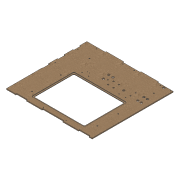
# Autodesk Inventor part: Lateral Derecho Carcasa
Saved by Autodesk Inventor 2020 (Build 240168000, 168)
## iProperties
Created: 2020-06-08
Part Number: Lateral Derecho Carcasa
Material: MDF Tablero de fibras de densidad media
Document SubType Name: Modeling
Designer: Pipi
Density: 0.8 g/cm^3
Appearance: Cartón - Ondulado
Mass: 1380.71 g
Surface Area: 4227.94 cm^2
Volume: 1725.88 cm^3
Author: Pipi
Autodesk Inventor part; units mm, degrees
ref_plane "YZ Plane" through (0, 0, 0) normal (1, 0, 0) x (0, 1, 0)
ref_plane "XZ Plane" through (0, 0, 0) normal (0, 1, 0) x (-1, 0, 0)
ref_plane "XY Plane" through (0, 0, 0) normal (0, 0, 1) x (1, 0, 0)
sketch "Boceto1" plane through (0, 0, 0) normal (0, 1, 0) x (-1, 0, 0)
  line L0 (31.3028, -81.5323) -> (31.3028, -546.5323)
  line L1 (526.8028, -376.5323) -> (521.3028, -376.5323)
  line L2 (521.3028, -326.5323) -> (526.8028, -326.5323)
  line L3 (116.3028, -128.5323) -> (116.3028, -344.5323)
  line L4 (398.303, -351.5323) -> (123.3028, -351.5323)
  line L5 (123.3028, -121.5323) -> (399.3028, -121.5323)
  line L6 (526.8028, -376.5323) -> (526.8028, -326.5323)
  line L7 (521.3028, -416.5323) -> (521.3028, -376.5323)
  line L8 (406.3028, -344.5323) -> (406.3028, -128.5323)
  line L9 (399.3028, -351.5323) -> (123.3028, -351.5323)
  line L10 (123.3028, -121.5323) -> (399.3028, -121.5323)
  arc A0 (399.3028, -351.5323) -> (406.3028, -344.5323) centre (399.3028, -344.5323) ccw
  arc A1 (406.3028, -128.5323) -> (399.3028, -121.5323) centre (399.3028, -128.5323) ccw
  arc A2 (123.3028, -121.5323) -> (116.3028, -128.5323) centre (123.3028, -128.5323) ccw
  arc A3 (116.3028, -344.5323) -> (123.3028, -351.5323) centre (123.3028, -344.5323) ccw
  line L11 (123.3028, -114.5323) -> (399.3028, -114.5323)
  line L12 (413.3028, -128.5323) -> (413.3028, -344.5323)
  line L13 (399.3028, -358.5323) -> (123.3028, -358.5323)
  line L14 (109.3028, -344.5323) -> (109.3028, -128.5323)
  line L15 (109.3028, -128.5323) -> (109.3028, -121.5323)
  line L16 (116.3028, -114.5323) -> (123.3028, -114.5323)
  line L17 (109.3028, -344.5323) -> (109.3028, -351.5323)
  line L18 (116.3028, -358.5323) -> (123.3028, -358.5323)
  line L19 (413.3028, -344.5323) -> (413.3028, -351.5323)
  line L20 (406.3028, -358.5323) -> (399.3028, -358.5323)
  line L21 (413.3028, -128.5323) -> (413.3028, -121.5323)
  line L22 (399.3028, -114.5323) -> (406.3028, -114.5323)
  arc A4 (413.3028, -121.5323) -> (406.3028, -114.5323) centre (406.3028, -121.5323) ccw
  arc A5 (406.3028, -358.5323) -> (413.3028, -351.5323) centre (406.3028, -351.5323) ccw
  arc A6 (109.3028, -351.5323) -> (116.3028, -358.5323) centre (116.3028, -351.5323) ccw
  arc A7 (116.3028, -114.5323) -> (109.3028, -121.5323) centre (116.3028, -121.5323) ccw
  line L23 (421.3028, -552.0323) -> (421.3028, -546.5323)
  line L24 (421.3028, -546.5323) -> (521.3028, -546.5323)
  line L25 (421.3028, -552.0323) -> (321.3028, -552.0323)
  line L26 (321.3028, -552.0323) -> (321.3028, -546.5323)
  line L27 (321.3028, -546.5323) -> (221.3028, -546.5323)
  line L28 (221.3028, -546.5323) -> (221.3028, -552.0323)
  line L29 (319.3028, -81.5323) -> (319.3028, -87.0323)
  line L30 (199.3028, -81.5323) -> (199.3028, -87.0323)
  line L31 (319.3028, -87.0323) -> (199.3028, -87.0323)
  circle A8 centre (76.3028, -156.5323) radius 3
  circle A9 centre (76.3028, -276.5323) radius 3
  line L32 (31.3028, -81.5323) -> (49.3028, -81.5323)
  circle A10 centre (76.3028, -481.0323) radius 3
  line L33 (521.3028, -81.5323) -> (523.8028, -81.5323)
  line L34 (523.8028, -81.5323) -> (523.8028, -286.5323)
  line L35 (523.8028, -286.5323) -> (521.3028, -286.5323)
  line L36 (521.3028, -286.5323) -> (521.3028, -326.5323)
  line L37 (221.3028, -552.0323) -> (121.3028, -552.0323)
  line L38 (121.3028, -552.0323) -> (121.3028, -546.5323)
  line L39 (121.3028, -546.5323) -> (31.3028, -546.5323)
  line L40 (526.8028, -416.5323) -> (521.3028, -416.5323)
  line L41 (526.8028, -416.5323) -> (526.8028, -466.5323)
  line L42 (526.8028, -466.5323) -> (521.3028, -466.5323)
  line L43 (521.3028, -466.5323) -> (521.3028, -506.5323)
  line L44 (521.3028, -506.5323) -> (526.8028, -506.5323)
  line L45 (526.8028, -546.5323) -> (526.8028, -506.5323)
  circle A11 centre (41.0178, -541.5323) radius 2
  circle A12 centre (349.1778, -378.6573) radius 2
  circle A13 centre (386.4278, -378.6573) radius 2
  circle A14 centre (367.8028, -383.8623) radius 2
  line L46 (261.3028, -358.5323) -> (261.3028, -396.5323)
  circle A15 centre (173.4278, -378.6573) radius 2
  circle A16 centre (136.1778, -378.6573) radius 2
  line L47 (521.3028, -546.5323) -> (526.8028, -546.5323)
  circle A17 centre (194.3028, -94.7473) radius 2
  circle A18 centre (324.3028, -94.7473) radius 2
  circle A19 centre (461.8028, -538.0323) radius 2
  circle A20 centre (311.8028, -538.0323) radius 2
  circle A21 centre (96.3028, -538.0323) radius 2
  circle A22 centre (246.3028, -538.0323) radius 2
  circle A23 centre (513.5878, -481.5323) radius 2
  circle A24 centre (513.5878, -351.5323) radius 2
  line L48 (319.3028, -81.5323) -> (409.3028, -81.5323)
  line L49 (409.3028, -81.5323) -> (409.3028, -87.0323)
  line L50 (409.3028, -87.0323) -> (469.3028, -87.0323)
  line L51 (469.3028, -87.0323) -> (469.3028, -81.5323)
  line L52 (521.3028, -81.5323) -> (469.3028, -81.5323)
  line L53 (409.3028, -81.5323) -> (319.3028, -81.5323)
  line L54 (199.3028, -81.5323) -> (109.3028, -81.5323)
  line L55 (109.3028, -81.5323) -> (109.3028, -87.0323)
  line L56 (109.3028, -87.0323) -> (49.3028, -87.0323)
  line L57 (49.3028, -87.0323) -> (49.3028, -81.5323)
  line L58 (31.3028, -81.5323) -> (49.3028, -81.5323)
  line L59 (109.3028, -81.5323) -> (199.3028, -81.5323)
  circle A25 centre (361.8028, -397.5323) radius 1.5
  circle A26 centre (373.8028, -397.5323) radius 1.5
  line L60 (81.3528, -532.0323) -> (70.2528, -532.0323)
  line L61 (70.2528, -532.0323) -> (70.2528, -542.7823)
  line L62 (70.2528, -542.7823) -> (81.3528, -542.7823)
  line L63 (81.3528, -542.7823) -> (81.3528, -532.0323)
  point P0 (0, 0)
  point P1 (398.3028, -355.6989)
  point P2 (109.3028, -358.5323)
  point P3 (413.3028, -358.5323)
  point P4 (413.3028, -114.5323)
  point P5 (398.303, -351.5323)
  dimension "d142" = 230
  dimension "d146" = 85
  dimension "d155" = 5.5
  dimension "d159" = 40
  dimension "d160" = 50
  dimension "d184" = 90
  dimension "d185" = 90
  dimension "d207" = 7
  dimension "d208" = 290
  dimension "d219" = 7
  dimension "d220" = 7
  dimension "d221" = 7
  dimension "d223" = 7
  dimension "d230" = 5.5
  dimension "d235" = 100
  dimension "d236" = 100
  dimension "d237" = 100
  dimension "d257" = 202
  dimension "d258" = 5.5
  dimension "d259" = 168
  dimension "d261" = 120
  dimension "d279" = 6
  dimension "d280" = 6
  dimension "d289" = 120
  dimension "d292" = 6
  dimension "d295" = 2.5
  dimension "d296" = 205
  dimension "d298" = 7
  dimension "d299" = 27.5
  dimension "d303" = 5.5
  dimension "d304" = 100
  dimension "d305" = 5.5
  dimension "d311" = 5.5
  dimension "d313" = 40
  dimension "d314" = 50
  dimension "d315" = 40
  dimension "d316" = 5.5
  dimension "d323" = 4
  dimension "d324" = 9.715
  dimension "d325" = 5
  dimension "d328" = 4
  dimension "d329" = 4
  dimension "d330" = 4
  dimension "d338" = 20.125
  dimension "d339" = 25.33
  dimension "d340" = 20.125
  dimension "d341" = 26.875
  dimension "d355" = 4
  dimension "d356" = 163
  dimension "d357" = 4
  dimension "d358" = 130
  dimension "d361" = 4
  dimension "d362" = 8.5
  dimension "d363" = 65
  dimension "d364" = 4
  dimension "d365" = 150
  dimension "d366" = 4
  dimension "d367" = 8.5
  dimension "d368" = 65
  dimension "d369" = 4
  dimension "d370" = 150
  dimension "d371" = 4
  dimension "d372" = 65
  dimension "d373" = 7.715
  constraints: 128 end point, 28 perpendicular, 27 centre point, 16 point on circle, 16 tangent, 11 horizontal, 10 point on line, 9 vertical, 6 equal radius, 3 parallel, 2 symmetric about line, 1 midpoint, 2 other
  measures "d142" distance between parallel lines of L4 L5
  measures "d146" distance between parallel lines of L0 L3
  measures "d155" distance between parallel lines of L7 L6
  measures "d159" distance of L7.start L1.end
  measures "d160" distance of L1.start L2.end
  measures "d184" angle of L2 L6
  measures "d185" angle of L1 L6
  measures "d207" radius of A0
  measures "d208" distance between parallel lines of L3 L8
  measures "d219" distance between parallel lines of L8 L12
  measures "d220" distance between parallel lines of L3 L14
  measures "d221" radius of A4
  measures "d223" distance between parallel lines of L4 L13
  measures "d230" distance of L23.start L23.end
  measures "d235" distance of L23.end L24.end
  measures "d236" distance of L23.start L25.end
  measures "d237" distance of L26.end L27.end
  measures "d257" distance of L33.start L29.start
  measures "d258" distance of L29.start L29.end
  measures "d259" distance of L0.start L30.start
  measures "d261" distance of L29.end L30.end
  measures "d279" diameter of A8
  measures "d280" diameter of A9
  measures "d289" distance of A8.centre A9.centre
  measures "d292" diameter of A10
  measures "d295" distance of L33.start L33.end
  measures "d296" distance of L33.end L34.end
  measures "d298" distance between parallel lines of L11 L5
  measures "d299" distance between parallel lines of L31 L11
  measures "d303" distance of L45.start L24.end
  measures "d304" distance of L28.end L37.end
  measures "d305" distance of L27.end L28.end
  measures "d311" distance of L37.end L38.end
  measures "d313" distance of L35.end L2.start
  measures "d314" distance of L40.start L41.end
  measures "d315" distance of L42.end L43.end
  measures "d316" distance of L43.end L44.end
  measures "d323" diameter of A11
  measures "d324" distance from line of L0 A11.centre
  measures "d325" distance from line of L39 A11.centre
  measures "d328" diameter of A12
  measures "d329" diameter of A13
  measures "d330" diameter of A14
  measures "d338" distance from line of L13 A13.centre
  measures "d339" distance from line of L13 A14.centre
  measures "d340" distance from line of L13 A12.centre
  measures "d341" distance from line of L19 A13.centre
  measures "d355" diameter of A17
  measures "d356" distance from line of L0 A17.centre
  measures "d357" diameter of A18
  measures "d358" distance of A17.centre A18.centre
  measures "d361" diameter of A19
  measures "d362" distance from line of L24 A19.centre
  measures "d363" distance from line of L45 A19.centre
  measures "d364" diameter of A20
  measures "d365" distance of A20.centre A19.centre
  measures "d366" diameter of A21
  measures "d367" distance from line of L39 A21.centre
  measures "d368" distance from line of L0 A21.centre
  measures "d369" diameter of A22
  measures "d370" distance of A21.centre A22.centre
  measures "d371" diameter of A23
  measures "d372" distance from line of L24 A23.centre
  measures "d373" distance from line of L43 A23.centre
extrude "Extrusión1" add sketch "Boceto1" along normal blind 5.5 contours L32 L57 L56 L55 L54 L30 L31 L29 L48 L49 L50 L51 L52 L33 L34 L35 L36 L2 L6 L1 L7 L40 L41 L42 L43 L44 L45 L47 L24 L23 L25 L26 L27 L28 L37 L38 L39 L0 | A14
extrude "Extrusión3" add sketch "Boceto1" along normal blind 2.5 contours L11 L22 A4 L21 L12 L19 A5 L20 L13 L18 A6 L17 L14 L15 A7 L16
sketch "Boceto2" plane through (0, 0, 0) normal (0, -1, 0) x (1, 0, 0)
  line L0 (-31.3028, -81.5323) -> (-31.3028, -546.5323) projected
  line L1 (-51.3028, -384.3323) -> (-51.3028, -448.8323)
  line L2 (-233.4894, -384.3323) -> (-51.3028, -384.3323)
  line L3 (-233.4894, -384.3323) -> (-310.8028, -384.3323)
  line L4 (-51.3028, -384.3323) -> (-51.3028, -448.8323)
  line L5 (-51.3028, -448.8323) -> (-310.8028, -448.8323)
  line L6 (-310.8028, -448.8323) -> (-310.8028, -384.3323)
  line L7 (-51.3028, -384.3323) -> (-51.3028, -409.3323)
  circle A0 centre (-177.3028, -408.8323) radius 6
  circle A1 centre (-294.3028, -408.8323) radius 6
  line L8 (-256.8028, -429.8323) -> (-256.8028, -387.8323)
  line L9 (-256.8028, -387.8323) -> (-214.8028, -387.8323)
  line L10 (-256.8028, -429.8323) -> (-214.8028, -429.8323)
  line L11 (-214.8028, -429.8323) -> (-214.8028, -387.8323)
  line L12 (-256.8028, -429.8323) -> (-256.8028, -424.3323)
  line L13 (-220.3028, -424.3323) -> (-220.3028, -393.3323)
  line L14 (-214.8028, -387.8323) -> (-214.8028, -393.3323)
  line L15 (-220.3028, -393.3323) -> (-251.3028, -393.3323)
  line L16 (-251.3028, -424.3323) -> (-251.3028, -393.3323)
  line L17 (-251.3028, -424.3323) -> (-220.3028, -424.3323)
  circle A2 centre (-251.3028, -424.3323) radius 4
  circle A3 centre (-251.3028, -393.3323) radius 4
  circle A4 centre (-220.3028, -424.3323) radius 4
  circle A5 centre (-220.3028, -393.3323) radius 4
  line L18 (-310.8028, -448.8323) -> (-310.8028, -443.8323)
  line L19 (-310.8028, -443.8323) -> (-298.3028, -443.8323)
  line L20 (-298.3028, -443.8323) -> (-273.3028, -443.8323)
  circle A6 centre (-298.3028, -443.8323) radius 6
  circle A7 centre (-273.3028, -443.8323) radius 6
  circle A8 centre (-66.3028, -433.8323) radius 6
  circle A9 centre (-86.3028, -433.8323) radius 6
  circle A10 centre (-86.3028, -398.8323) radius 6
  circle A11 centre (-66.3028, -398.8323) radius 6
  line L21 (-235.8028, -429.8323) -> (-235.8028, -387.8323)
  line L22 (-256.8028, -408.8323) -> (-214.8028, -408.8323)
  line L23 (-399.3028, -351.5323) -> (-123.3028, -351.5323) projected
  circle A12 centre (-131.3028, -430.8323) radius 3
  circle A13 centre (-131.3028, -402.3323) radius 3
  circle A14 centre (-275.8028, -416.8323) radius 3
  point P0 (0, 0)
  point P1 (-31.3028, -85.6989)
  point P2 (-521.3028, -627.1989)
  point P3 (-31.3028, -532.1989)
  dimension "d68" = 64.5
  dimension "d69" = 259.5
  dimension "d70" = 20
  dimension "d71" = 25
  dimension "d73" = 12
  dimension "d75" = 12
  dimension "d76" = 126
  dimension "d77" = 243
  dimension "d78" = 42
  dimension "d79" = 42
  dimension "d80" = 5.5
  dimension "d82" = 5.5
  dimension "d83" = 5.5
  dimension "d84" = 8
  dimension "d85" = 8
  dimension "d86" = 8
  dimension "d87" = 8
  dimension "d88" = 3.5
  dimension "d91" = 5
  dimension "d92" = 12.5
  dimension "d93" = 25
  dimension "d94" = 12
  dimension "d95" = 12
  dimension "d96" = 12
  dimension "d97" = 12
  dimension "d98" = 12
  dimension "d99" = 12
  dimension "d102" = 20
  dimension "d103" = 15
  dimension "d106" = 20
  dimension "d107" = 15
  dimension "d148" = 58.5
  dimension "d193" = 5.5
  dimension "d194" = 5.5
  dimension "d213" = 35
  dimension "d214" = 35
  dimension "d263" = 6
  dimension "d264" = 6
  dimension "d269" = 6
  dimension "d273" = 18
  dimension "d274" = 18
  dimension "d275" = 32
  dimension "d300" = 90
  dimension "d301" = 32.8
  dimension "d383" = 40
  dimension "d384" = 40
  dimension "d385" = 15
  dimension "d386" = 15
  constraints: 44 end point, 15 centre point, 9 perpendicular, 6 coincident, 5 point on line, 4 midpoint, 2 horizontal, 2 vertical
  measures "d68" distance of L1.end L1.start
  measures "d69" distance of L1.end L5.end
  measures "d70" distance between parallel lines of L0 L1
  measures "d71" distance of L1.start L7.end
  measures "d73" diameter of A0
  measures "d75" diameter of A1
  measures "d76" distance from line of L7 A0.centre
  measures "d77" distance from line of A1.centre L1
  measures "d78" distance of L8.start L8.end
  measures "d79" distance of L8.end L9.end
  measures "d80" distance of L8.start L12.end
  measures "d82" distance of L9.end L14.end
  measures "d83" distance of L16.start L12.end
  measures "d84" diameter of A2
  measures "d85" diameter of A3
  measures "d86" diameter of A4
  measures "d87" diameter of A5
  measures "d88" distance between parallel lines of L3 L9
  measures "d91" distance of L5.end L18.end
  measures "d92" distance of L18.end L19.end
  measures "d93" distance of L19.end L20.end
  measures "d94" diameter of A6
  measures "d95" diameter of A7
  measures "d96" diameter of A8
  measures "d97" diameter of A9
  measures "d98" diameter of A10
  measures "d99" diameter of A11
  measures "d102" distance of A9.centre A8.centre
  measures "d103" distance from line of L1 A8.centre
  measures "d106" distance of A11.centre A10.centre
  measures "d107" distance from line of L7 A11.centre
  measures "d148" distance from line of A0.centre L21
  measures "d193" distance between parallel lines of L9 L15
  measures "d194" distance between parallel lines of L10 L17
  measures "d213" distance of A11.centre A8.centre
  measures "d214" distance of A10.centre A9.centre
  measures "d263" diameter of A12
  measures "d264" diameter of A13
  measures "d269" diameter of A14
  measures "d273" distance from line of L5 A12.centre
  measures "d274" distance from line of L2 A13.centre
  measures "d275" distance from line of L5 A14.centre
  measures "d300" angle of L2 L1
  measures "d301" distance between parallel lines of L23 L2
  measures "d383" distance from line of L5 A1.centre
  measures "d384" distance from line of L5 A0.centre
  measures "d385" distance from line of L5 A9.centre
  measures "d386" distance from line of L5 A8.centre
sketch "Boceto3" plane through (0, 5.5, 0) normal (0, 1, 0) x (1, 0, 0)
  circle A0 centre (-434.9448, 139.5323) radius 3
  circle A1 centre (-434.9448, 304.5323) radius 3
  circle A2 centre (-434.9448, 469.5323) radius 3
  line L0 (-523.8028, 286.5323) -> (-523.8028, 81.5323) projected
  line L1 (-523.8028, 81.5323) -> (-469.3028, 81.5323) projected
  line L2 (-521.3028, 326.5323) -> (-521.3028, 286.5323) projected
  line L3 (-521.3028, 506.5323) -> (-521.3028, 466.5323) projected
  point P0 (0, 0)
  point P1 (-319.3028, 81.5323)
  dimension "d167" = 6
  dimension "d168" = 6
  dimension "d169" = 6
  dimension "d317" = 88.858
  dimension "d318" = 165
  dimension "d319" = 165
  dimension "d320" = 58
  dimension "d321" = 86.358
  dimension "d322" = 86.358
  constraints: 3 centre point
  measures "d167" diameter of A0
  measures "d168" diameter of A1
  measures "d169" diameter of A2
  measures "d317" distance from line of L0 A0.centre
  measures "d318" distance of A1.centre A0.centre
  measures "d319" distance of A2.centre A1.centre
  measures "d320" distance from line of L1 A0.centre
  measures "d321" distance from line of L2 A1.centre
  measures "d322" distance from line of L3 A2.centre
extrude "Extrusión5" cut sketch "Boceto3" against normal blind 10
extrude "Extrusión6" cut sketch "Boceto2" against normal blind 10 contours A7 L5 | L5 A7 | A6 L20 L19 | L19 L20 A6 L5 | A6 L5 | A0 | A1 | A2 L16 L17 | L17 L16 A2 | A4 L13 L17 | L17 L13 A4 | A3 L15 L16 | L16 L15 A3 | A5 L15 L13 | L13 L15 A5 | A8 | A9 | A10 | A11 | A12 | A13 | A14
